Autodesk Inventor part; units mm, degrees
(part 2 of 2)
sketch "スケッチ11" plane through (0, 0, 1) normal (0, 0, 1) x (1, 0, 0)
  circle A0 centre (-32.2184, -15.8179) radius 1.1 projected
  circle A1 centre (-126.8791, -41.1821) radius 1.1 projected
  line L0 (-129.0618, -44.3889) -> (-95.4376, -78.0131) projected
  arc A2 (-94.0487, -79.9174) -> (-95.4376, -78.0131) centre (-96.0487, -79.9174) ccw projected
  line L1 (-94.0487, -79.9174) -> (-94.0487, -93) projected
  arc A3 (-96.0487, -95) -> (-94.0487, -93) centre (-96.0487, -93) ccw projected
  line L2 (-96.0487, -95) -> (-105.7028, -95) projected
  arc A4 (-105.7028, -95) -> (-107.2443, -95.7258) centre (-105.7028, -97) ccw projected
  line L3 (-107.2443, -95.7258) -> (-113.0806, -102.7869) projected
  arc A5 (-115.4882, -103.3155) -> (-113.0806, -102.7869) centre (-114.6222, -101.5127) ccw projected
  arc A6 (-154.3642, -64.4395) -> (-115.4882, -103.3155) centre (-79.5487, -28.5) ccw projected
  arc A7 (-153.8356, -62.0319) -> (-154.3642, -64.4395) centre (-152.5614, -63.5735) ccw projected
  line L4 (-153.8356, -62.0319) -> (-146.7745, -56.1956) projected
  arc A8 (-146.7745, -56.1956) -> (-146.0487, -54.654) centre (-148.0487, -54.654) ccw projected
  line L5 (-146.0487, -54.654) -> (-146.0487, -45) projected
  arc A9 (-144.0487, -43) -> (-146.0487, -45) centre (-144.0487, -45) ccw projected
  line L6 (-144.0487, -43) -> (-130.9661, -43) projected
  arc A10 (-129.0618, -44.3889) -> (-130.9661, -43) centre (-130.9661, -45) ccw projected
  line L7 (-30.0357, -12.6111) -> (-63.6598, 21.0131) projected
  arc A11 (-65.0487, 22.9174) -> (-63.6598, 21.0131) centre (-63.0487, 22.9174) ccw projected
  line L8 (-65.0487, 22.9174) -> (-65.0487, 36) projected
  arc A12 (-63.0487, 38) -> (-65.0487, 36) centre (-63.0487, 36) ccw projected
  line L9 (-63.0487, 38) -> (-53.3947, 38) projected
  arc A13 (-53.3947, 38) -> (-51.8531, 38.7258) centre (-53.3947, 40) ccw projected
  line L10 (-51.8531, 38.7258) -> (-46.0168, 45.7869) projected
  arc A14 (-43.6092, 46.3155) -> (-46.0168, 45.7869) centre (-44.4752, 44.5127) ccw projected
  arc A15 (-4.7333, 7.4395) -> (-43.6092, 46.3155) centre (-79.5487, -28.5) ccw projected
  arc A16 (-5.2619, 5.0319) -> (-4.7333, 7.4395) centre (-6.5361, 6.5735) ccw projected
  line L11 (-5.2619, 5.0319) -> (-12.3229, -0.8044) projected
  arc A17 (-12.3229, -0.8044) -> (-13.0487, -2.346) centre (-11.0487, -2.346) ccw projected
  line L12 (-13.0487, -2.346) -> (-13.0487, -12) projected
  arc A18 (-15.0487, -14) -> (-13.0487, -12) centre (-15.0487, -12) ccw projected
  line L13 (-15.0487, -14) -> (-28.1313, -14) projected
  arc A19 (-30.0357, -12.6111) -> (-28.1313, -14) centre (-28.1313, -12) ccw projected
  circle A20 centre (-118.4396, -24.9645) radius 1.1 projected
  circle A21 centre (-40.6579, -32.0355) radius 1.1 projected
  circle A22 centre (-76.0132, -67.3909) radius 1.1 projected
  circle A23 centre (-83.0843, 10.3909) radius 1.1 projected
  circle A24 centre (-89.0947, -67.7444) radius 1.1 projected
  circle A25 centre (-118.7932, -38.0459) radius 1.1 projected
  circle A26 centre (-40.3043, -18.9541) radius 1.1 projected
  circle A27 centre (-70.0028, 10.7444) radius 1.1 projected
  line L14 (-17.4123, -55.2811) -> (-3.6474, -69.046) projected
  arc A28 (-3.6474, -69.046) -> (-1.2521, -68.6701) centre (-2.5867, -67.9854) ccw projected
  arc A29 (-1.2521, -68.6701) -> (4.2199, -55.4595) centre (-79.5487, -28.5) ccw projected
  arc A30 (4.2199, -55.4595) -> (2.792, -53.5) centre (2.792, -55) ccw projected
  line L15 (2.792, -53.5) -> (-6.0487, -53.5) projected
  arc A31 (-8.0487, -51.5) -> (-6.0487, -53.5) centre (-6.0487, -51.5) ccw projected
  line L16 (-8.0487, -51.5) -> (-8.0487, -5.5) projected
  arc A32 (-6.0487, -3.5) -> (-8.0487, -5.5) centre (-6.0487, -5.5) ccw projected
  line L17 (-6.0487, -3.5) -> (2.792, -3.5) projected
  arc A33 (2.792, -3.5) -> (4.2199, -1.5405) centre (2.792, -2) ccw projected
  arc A34 (4.2199, -1.5405) -> (-52.5892, 55.2686) centre (-79.5487, -28.5) ccw projected
  arc A35 (-52.5892, 55.2686) -> (-54.5487, 53.8408) centre (-53.0487, 53.8408) ccw projected
  line L18 (-54.5487, 53.8408) -> (-54.5487, 45) projected
  arc A36 (-56.5487, 43) -> (-54.5487, 45) centre (-56.5487, 45) ccw projected
  line L19 (-56.5487, 43) -> (-102.5487, 43) projected
  arc A37 (-104.5487, 45) -> (-102.5487, 43) centre (-102.5487, 45) ccw projected
  line L20 (-104.5487, 45) -> (-104.5487, 53.8408) projected
  arc A38 (-104.5487, 53.8408) -> (-106.5083, 55.2686) centre (-106.0487, 53.8408) ccw projected
  arc A39 (-106.5083, 55.2686) -> (-119.7188, 49.7966) centre (-79.5487, -28.5) ccw projected
  arc A40 (-119.7188, 49.7966) -> (-120.0948, 47.4014) centre (-119.0341, 48.462) ccw projected
  line L21 (-120.0948, 47.4014) -> (-106.3298, 33.6364) projected
  arc A41 (-106.3298, 30.808) -> (-106.3298, 33.6364) centre (-107.744, 32.2222) ccw projected
  line L22 (-138.8567, -1.7189) -> (-106.3298, 30.808) projected
  arc A42 (-141.6851, -1.7189) -> (-138.8567, -1.7189) centre (-140.2709, -0.3047) ccw projected
  line L23 (-141.6851, -1.7189) -> (-155.4501, 12.046) projected
  arc A43 (-155.4501, 12.046) -> (-157.8454, 11.6701) centre (-156.5108, 10.9854) ccw projected
  arc A44 (-157.8454, 11.6701) -> (-163.3174, -1.5405) centre (-79.5487, -28.5) ccw projected
  arc A45 (-163.3174, -1.5405) -> (-161.8895, -3.5) centre (-161.8895, -2) ccw projected
  line L24 (-161.8895, -3.5) -> (-153.0487, -3.5) projected
  arc A46 (-151.0487, -5.5) -> (-153.0487, -3.5) centre (-153.0487, -5.5) ccw projected
  line L25 (-151.0487, -5.5) -> (-151.0487, -51.5) projected
  arc A47 (-153.0487, -53.5) -> (-151.0487, -51.5) centre (-153.0487, -51.5) ccw projected
  line L26 (-153.0487, -53.5) -> (-161.8895, -53.5) projected
  arc A48 (-161.8895, -53.5) -> (-163.3174, -55.4595) centre (-161.8895, -55) ccw projected
  arc A49 (-163.3174, -55.4595) -> (-106.5083, -112.2686) centre (-79.5487, -28.5) ccw projected
  arc A50 (-106.5083, -112.2686) -> (-104.5487, -110.8408) centre (-106.0487, -110.8408) ccw projected
  line L27 (-104.5487, -110.8408) -> (-104.5487, -102) projected
  arc A51 (-102.5487, -100) -> (-104.5487, -102) centre (-102.5487, -102) ccw projected
  line L28 (-102.5487, -100) -> (-56.5487, -100) projected
  arc A52 (-54.5487, -102) -> (-56.5487, -100) centre (-56.5487, -102) ccw projected
  line L29 (-54.5487, -102) -> (-54.5487, -110.8408) projected
  arc A53 (-54.5487, -110.8408) -> (-52.5892, -112.2686) centre (-53.0487, -110.8408) ccw projected
  arc A54 (-52.5892, -112.2686) -> (-39.3786, -106.7966) centre (-79.5487, -28.5) ccw projected
  arc A55 (-39.3786, -106.7966) -> (-39.0027, -104.4014) centre (-40.0634, -105.462) ccw projected
  line L30 (-39.0027, -104.4014) -> (-52.7676, -90.6364) projected
  arc A56 (-52.7676, -87.808) -> (-52.7676, -90.6364) centre (-51.3534, -89.2222) ccw projected
  line L31 (-20.2407, -55.2811) -> (-52.7676, -87.808) projected
  arc A57 (-17.4123, -55.2811) -> (-20.2407, -55.2811) centre (-18.8265, -56.6953) ccw projected
  circle A58 centre (-88.0487, -96.5) radius 0.8 projected
  circle A59 centre (-71.0487, -96.5) radius 0.8 projected
  circle A60 centre (-159.0975, -57) radius 1.3 projected
  circle A61 centre (-108.0487, -108.0487) radius 1.3 projected
  circle A62 centre (0, 0) radius 1.3 projected
  circle A63 centre (-11.5487, -37) radius 0.8 projected
  circle A64 centre (-11.5487, -20) radius 0.8 projected
  circle A65 centre (-71.0487, 39.5) radius 0.8 projected
  circle A66 centre (-88.0487, 39.5) radius 0.8 projected
  circle A67 centre (-147.5487, -20) radius 0.8 projected
  circle A68 centre (-147.5487, -37) radius 0.8 projected
  circle A69 centre (-51.0487, 51.0487) radius 1.3 projected
  circle A70 centre (-32.2184, -15.8179) radius 3
  circle A71 centre (-126.8791, -41.1821) radius 3
  point P0 (0, 0)
  dimension "d90" = 6
  constraints: 2 centre point, 2 coincident, 1 equal radius
  measures "d90" diameter of A71
extrude "押し出し12" add sketch "スケッチ11" along normal blind 4 contours A70 | A71
fillet "フィレット4" radius 2 2 edges at (-129.8791, -41.1821, 1) (-35.2184, -15.8179, 1)
sketch "スケッチ13" plane through (0, 0, -2) normal (0, 0, -1) x (-1, 0, 0)
  circle A0 centre (152.6453, 4.2915) radius 1 projected
  circle A1 centre (152.6453, 4.2915) radius 1 projected
  circle A2 centre (112.3402, 44.5966) radius 1 projected
  circle A3 centre (46.7572, -101.5966) radius 1 projected
  circle A4 centre (6.4522, -61.2915) radius 1 projected
  point P0 (0, 0)
extrude "押し出し13" cut sketch "スケッチ13" against normal up to surface (3 mm away)
sketch "スケッチ14" plane through (0, 0, 1) normal (0, 0, 1) x (1, 0, 0)
  circle A0 centre (-46.7572, -101.5966) radius 1 projected
  circle A1 centre (-152.6453, 4.2915) radius 1 projected
  circle A2 centre (-6.4522, -61.2915) radius 1 projected
  circle A3 centre (-112.3402, 44.5966) radius 1 projected
  arc A4 (-31.8124, -10.8344) -> (-27.5605, -14) centre (-32.2184, -15.8179) ccw projected
  line L0 (-31.8124, -10.8344) -> (-63.6598, 21.0131) projected
  arc A5 (-65.0487, 22.9174) -> (-63.6598, 21.0131) centre (-63.0487, 22.9174) ccw projected
  line L1 (-65.0487, 22.9174) -> (-65.0487, 36) projected
  arc A6 (-63.0487, 38) -> (-65.0487, 36) centre (-63.0487, 36) ccw projected
  line L2 (-63.0487, 38) -> (-53.3947, 38) projected
  arc A7 (-53.3947, 38) -> (-51.8531, 38.7258) centre (-53.3947, 40) ccw projected
  line L3 (-51.8531, 38.7258) -> (-46.0168, 45.7869) projected
  arc A8 (-43.6092, 46.3155) -> (-46.0168, 45.7869) centre (-44.4752, 44.5127) ccw projected
  arc A9 (-4.7333, 7.4395) -> (-43.6092, 46.3155) centre (-79.5487, -28.5) ccw projected
  arc A10 (-5.2619, 5.0319) -> (-4.7333, 7.4395) centre (-6.5361, 6.5735) ccw projected
  line L4 (-5.2619, 5.0319) -> (-12.3229, -0.8044) projected
  arc A11 (-12.3229, -0.8044) -> (-13.0487, -2.346) centre (-11.0487, -2.346) ccw projected
  line L5 (-13.0487, -2.346) -> (-13.0487, -12) projected
  arc A12 (-15.0487, -14) -> (-13.0487, -12) centre (-15.0487, -12) ccw projected
  line L6 (-15.0487, -14) -> (-27.5605, -14) projected
  arc A13 (-127.2851, -46.1656) -> (-131.5369, -43) centre (-126.8791, -41.1821) ccw projected
  line L7 (-127.2851, -46.1656) -> (-95.4376, -78.0131) projected
  arc A14 (-94.0487, -79.9174) -> (-95.4376, -78.0131) centre (-96.0487, -79.9174) ccw projected
  line L8 (-94.0487, -79.9174) -> (-94.0487, -93) projected
  arc A15 (-96.0487, -95) -> (-94.0487, -93) centre (-96.0487, -93) ccw projected
  line L9 (-96.0487, -95) -> (-105.7028, -95) projected
  arc A16 (-105.7028, -95) -> (-107.2443, -95.7258) centre (-105.7028, -97) ccw projected
  line L10 (-107.2443, -95.7258) -> (-113.0806, -102.7869) projected
  arc A17 (-115.4882, -103.3155) -> (-113.0806, -102.7869) centre (-114.6222, -101.5127) ccw projected
  arc A18 (-154.3642, -64.4395) -> (-115.4882, -103.3155) centre (-79.5487, -28.5) ccw projected
  arc A19 (-153.8356, -62.0319) -> (-154.3642, -64.4395) centre (-152.5614, -63.5735) ccw projected
  line L11 (-153.8356, -62.0319) -> (-146.7745, -56.1956) projected
  arc A20 (-146.7745, -56.1956) -> (-146.0487, -54.654) centre (-148.0487, -54.654) ccw projected
  line L12 (-146.0487, -54.654) -> (-146.0487, -45) projected
  arc A21 (-144.0487, -43) -> (-146.0487, -45) centre (-144.0487, -45) ccw projected
  line L13 (-144.0487, -43) -> (-131.5369, -43) projected
  circle A22 centre (-118.4396, -24.9645) radius 1.1 projected
  circle A23 centre (-40.6579, -32.0355) radius 1.1 projected
  circle A24 centre (-76.0132, -67.3909) radius 1.1 projected
  circle A25 centre (-83.0843, 10.3909) radius 1.1 projected
  circle A26 centre (-89.0947, -67.7444) radius 1.1 projected
  circle A27 centre (-118.7932, -38.0459) radius 1.1 projected
  circle A28 centre (-40.3043, -18.9541) radius 1.1 projected
  circle A29 centre (-70.0028, 10.7444) radius 1.1 projected
  line L14 (-17.4123, -55.2811) -> (-3.6474, -69.046) projected
  arc A30 (-3.6474, -69.046) -> (-1.2521, -68.6701) centre (-2.5867, -67.9854) ccw projected
  arc A31 (-1.2521, -68.6701) -> (4.2199, -55.4595) centre (-79.5487, -28.5) ccw projected
  arc A32 (4.2199, -55.4595) -> (2.792, -53.5) centre (2.792, -55) ccw projected
  line L15 (2.792, -53.5) -> (-6.0487, -53.5) projected
  arc A33 (-8.0487, -51.5) -> (-6.0487, -53.5) centre (-6.0487, -51.5) ccw projected
  line L16 (-8.0487, -51.5) -> (-8.0487, -5.5) projected
  arc A34 (-6.0487, -3.5) -> (-8.0487, -5.5) centre (-6.0487, -5.5) ccw projected
  line L17 (-6.0487, -3.5) -> (2.792, -3.5) projected
  arc A35 (2.792, -3.5) -> (4.2199, -1.5405) centre (2.792, -2) ccw projected
  arc A36 (4.2199, -1.5405) -> (-52.5892, 55.2686) centre (-79.5487, -28.5) ccw projected
  arc A37 (-52.5892, 55.2686) -> (-54.5487, 53.8408) centre (-53.0487, 53.8408) ccw projected
  line L18 (-54.5487, 53.8408) -> (-54.5487, 45) projected
  arc A38 (-56.5487, 43) -> (-54.5487, 45) centre (-56.5487, 45) ccw projected
  line L19 (-56.5487, 43) -> (-102.5487, 43) projected
  arc A39 (-104.5487, 45) -> (-102.5487, 43) centre (-102.5487, 45) ccw projected
  line L20 (-104.5487, 45) -> (-104.5487, 53.8408) projected
  arc A40 (-104.5487, 53.8408) -> (-106.5083, 55.2686) centre (-106.0487, 53.8408) ccw projected
  arc A41 (-106.5083, 55.2686) -> (-119.7188, 49.7966) centre (-79.5487, -28.5) ccw projected
  arc A42 (-119.7188, 49.7966) -> (-120.0948, 47.4014) centre (-119.0341, 48.462) ccw projected
  line L21 (-120.0948, 47.4014) -> (-106.3298, 33.6364) projected
  arc A43 (-106.3298, 30.808) -> (-106.3298, 33.6364) centre (-107.744, 32.2222) ccw projected
  line L22 (-138.8567, -1.7189) -> (-106.3298, 30.808) projected
  arc A44 (-141.6851, -1.7189) -> (-138.8567, -1.7189) centre (-140.2709, -0.3047) ccw projected
  line L23 (-141.6851, -1.7189) -> (-155.4501, 12.046) projected
  arc A45 (-155.4501, 12.046) -> (-157.8454, 11.6701) centre (-156.5108, 10.9854) ccw projected
  arc A46 (-157.8454, 11.6701) -> (-163.3174, -1.5405) centre (-79.5487, -28.5) ccw projected
  arc A47 (-163.3174, -1.5405) -> (-161.8895, -3.5) centre (-161.8895, -2) ccw projected
  line L24 (-161.8895, -3.5) -> (-153.0487, -3.5) projected
  arc A48 (-151.0487, -5.5) -> (-153.0487, -3.5) centre (-153.0487, -5.5) ccw projected
  line L25 (-151.0487, -5.5) -> (-151.0487, -51.5) projected
  arc A49 (-153.0487, -53.5) -> (-151.0487, -51.5) centre (-153.0487, -51.5) ccw projected
  line L26 (-153.0487, -53.5) -> (-161.8895, -53.5) projected
  arc A50 (-161.8895, -53.5) -> (-163.3174, -55.4595) centre (-161.8895, -55) ccw projected
  arc A51 (-163.3174, -55.4595) -> (-106.5083, -112.2686) centre (-79.5487, -28.5) ccw projected
  arc A52 (-106.5083, -112.2686) -> (-104.5487, -110.8408) centre (-106.0487, -110.8408) ccw projected
  line L27 (-104.5487, -110.8408) -> (-104.5487, -102) projected
  arc A53 (-102.5487, -100) -> (-104.5487, -102) centre (-102.5487, -102) ccw projected
  line L28 (-102.5487, -100) -> (-56.5487, -100) projected
  arc A54 (-54.5487, -102) -> (-56.5487, -100) centre (-56.5487, -102) ccw projected
  line L29 (-54.5487, -102) -> (-54.5487, -110.8408) projected
  arc A55 (-54.5487, -110.8408) -> (-52.5892, -112.2686) centre (-53.0487, -110.8408) ccw projected
  arc A56 (-52.5892, -112.2686) -> (-39.3786, -106.7966) centre (-79.5487, -28.5) ccw projected
  arc A57 (-39.3786, -106.7966) -> (-39.0027, -104.4014) centre (-40.0634, -105.462) ccw projected
  line L30 (-39.0027, -104.4014) -> (-52.7676, -90.6364) projected
  arc A58 (-52.7676, -87.808) -> (-52.7676, -90.6364) centre (-51.3534, -89.2222) ccw projected
  line L31 (-20.2407, -55.2811) -> (-52.7676, -87.808) projected
  arc A59 (-17.4123, -55.2811) -> (-20.2407, -55.2811) centre (-18.8265, -56.6953) ccw projected
  circle A60 centre (-88.0487, -96.5) radius 0.8 projected
  circle A61 centre (-71.0487, -96.5) radius 0.8 projected
  circle A62 centre (-159.0975, -57) radius 1.3 projected
  circle A63 centre (-108.0487, -108.0487) radius 1.3 projected
  circle A64 centre (0, 0) radius 1.3 projected
  circle A65 centre (-11.5487, -37) radius 0.8 projected
  circle A66 centre (-11.5487, -20) radius 0.8 projected
  circle A67 centre (-71.0487, 39.5) radius 0.8 projected
  circle A68 centre (-88.0487, 39.5) radius 0.8 projected
  circle A69 centre (-147.5487, -20) radius 0.8 projected
  circle A70 centre (-147.5487, -37) radius 0.8 projected
  circle A71 centre (-51.0487, 51.0487) radius 1.3 projected
  line L32 (-48.9031, 53.9915) -> (2.9428, 2.1456)
  line L33 (-31.8124, -10.8344) -> (-63.6598, 21.0131) projected
  line L34 (-162.0402, -59.1456) -> (-110.1943, -110.9915)
  line L35 (-122.5933, 14.5445) -> (-36.5042, -71.5445)
  point P0 (0, 0)
  point P1 (-7.3437, 12.432)
  point P2 (-38.6167, 43.705)
  point P3 (-120.4808, -100.705)
  point P4 (-151.7538, -69.432)
  dimension "d96" = 80
  constraints: 6 end point, 4 point on circle, 2 midpoint, 2 parallel, 1 other
  measures "d96" distance between parallel lines of L35 L32
extrude "押し出し14" [suppressed]
equation "\"d5\" = d4"
equation "\"d7\" = d6"
equation "\"d8\" = d9"
equation "\"d20\" = d19"
equation "\"d41\" = d39"
